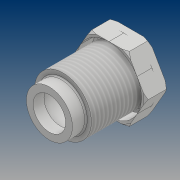
# Autodesk Inventor part: MUSAB2
Saved by Autodesk Inventor 2021 (Build 250183000, 183)
## iProperties
Created: 2017-09-12
Part Number: MUSAB2
Material: Generic
Document SubType Name: Modeling
Designer: Amer Mohia
Density: 1 g/cm^3
Appearance: Default
Author: Amer Mohia
Autodesk Inventor part; units mm, degrees
ref_plane "YZ Plane" through (0, 0, 0) normal (1, 0, 0) x (0, 1, 0)
ref_plane "XZ Plane" through (0, 0, 0) normal (0, 1, 0) x (-1, 0, 0)
sketch "Sketch1" plane through (0, 0, 0) normal (0, 0, 1) x (1, 0, 0)
  line L0 (-7.9743, 17.1273) -> (-7.9743, -10.9738)
  line L1 (4.0257, 11.5) -> (4.0257, 9)
  line L2 (4.0257, 9) -> (2.5257, 9)
  line L3 (2.5257, 9) -> (2.5257, -13.5)
  line L4 (2.5257, -13.5) -> (0.5257, -13.5)
  line L5 (0.5257, -13.5) -> (0.5257, -18.5)
  line L6 (4.0257, 11.5) -> (0.5257, 11.5)
  line L7 (0.5257, 11.5) -> (0.5257, 6.5)
  line L8 (0.5257, -2.5) -> (-0.9743, -2.5)
  line L9 (-0.9743, -2.5) -> (-0.9743, -11.3304)
  line L10 (-1.9743, -14.5) -> (-1.9743, -18.5)
  line L11 (-1.9743, -18.5) -> (0.5257, -18.5)
  line L12 (-1.9743, -14.5) -> (-0.9743, -14.5)
  line L13 (-0.9743, -14.5) -> (-0.9743, -11.3304)
  line L14 (0.0257, 6.5) -> (0.0257, 0)
  line L15 (0.5257, 6.5) -> (0.0257, 6.5)
  line L16 (0.0257, 0) -> (0.3257, 0)
  line L17 (0.8257, -0.5) -> (0.8257, -2.5)
  line L18 (0.8257, -2.5) -> (0.5257, -2.5)
  arc A0 (0.8257, -0.5) -> (0.3257, 0) centre (0.3257, -0.5) ccw
  point P0 (0.8257, 0)
  dimension "d6" = 14
  dimension "d7" = 17
  dimension "d8" = 21
  dimension "d10" = 5
  dimension "d11" = 12
  dimension "d12" = 4
  dimension "d13" = 30
  dimension "d14" = 5
  dimension "d18" = 24
  dimension "d19" = 16
  dimension "d20" = 17
  dimension "d21" = 0.8
  dimension "d22" = 2.5
  dimension "d23" = 0.5
  constraints: 38 end point, 8 perpendicular, 5 horizontal, 4 vertical, 3 point on line, 2 point on circle, 2 tangent, 1 centre point
  measures "d6" diameter of L9 L0
  measures "d7" diameter of L5 L0
  measures "d8" diameter of L3 L0
  measures "d10" distance of L4.end L5.end
  measures "d11" diameter of L10 L0
  measures "d12" distance of L10.start L10.end
  measures "d13" distance between parallel lines of L11 L6
  measures "d14" distance of L6.end L7.end
  measures "d18" diameter of L1 L0
  measures "d19" diameter of L14 L0
  measures "d20" diameter of L7 L0
  measures "d21" distance of L14.end point (0.826, 0)
  measures "d22" distance of point (0.826, 0) L17.end
  measures "d23" radius of A0
revolve "Revolution1" add sketch "Sketch1" angle 360 about axis through (-7.9743, 17.1273, 0) along (0, -1, 0)
sketch "Sketch2" plane through (-7.9743, 11.5, 0) normal (0, 1, 0) x (1, 0, 0)
  circle A0 centre (0, 0) radius 12 projected
  line L0 (6.9282, 12) -> (13.8564, 0)
  line L1 (13.8564, 0) -> (6.9282, -12)
  line L2 (6.9282, -12) -> (-6.9282, -12)
  line L3 (-6.9282, -12) -> (-13.8564, 0)
  line L4 (-13.8564, 0) -> (-6.9282, 12)
  line L5 (-6.9282, 12) -> (6.9282, 12)
  point P0 (7.9743, 0)
  point P1 (0, 12)
  constraints: 12 end point, 1 midpoint, 1 vertical alignment, 14 other
extrude "Extrusion1" add sketch "Sketch2" against normal blind 8 contours A0 L0 L1 | A0 L5 L0 | L1 L2 A0 | A0 L4 L5 | L2 L3 A0 | A0 L3 L4
sketch "Sketch3" plane through (0, 0, 0) normal (0, 0, 1) x (1, 0, 0)
  line L0 (2.418, 3.5) -> (5.8821, 3.5) projected
  line L1 (-1.0461, 11.5) -> (-1.0461, 3.5) projected
  line L2 (-1.0461, 11.5) -> (5.8821, 11.5) projected
  line L3 (5.8821, 11.5) -> (5.8821, 3.5) projected
  line L4 (-21.8307, 3.5) -> (-18.3666, 3.5) projected
  line L5 (-21.8307, 11.5) -> (-21.8307, 3.5) projected
  line L6 (-21.8307, 11.5) -> (-14.9025, 11.5) projected
  line L7 (-14.9025, 11.5) -> (-14.9025, 3.5) projected
  line L8 (-7.9743, 20.7963) -> (-7.9743, 13.4843)
  line L9 (6.3821, 12) -> (4.1894, 12)
  line L10 (6.3821, 12) -> (6.3821, 10.5)
  line L11 (4.1894, 12) -> (6.3821, 10.5)
  line L12 (-18.3666, 9) -> (-18.3666, 3.5) projected
  line L13 (-18.3666, 3.5) -> (-14.9025, 3.5) projected
  line L14 (2.418, 9) -> (2.418, 3.5) projected
  line L15 (-1.0461, 3.5) -> (2.418, 3.5) projected
  point P0 (0, 0)
  dimension "d36" = 0.5
  dimension "d38" = 0.5
  dimension "d39" = 1.5
  constraints: 8 end point, 2 vertical, 1 horizontal
  measures "d36" distance between parallel lines of L3 L10
  measures "d38" distance between parallel lines of L2 L9
  measures "d39" distance of L9.start L10.end
revolve "Revolution2" cut sketch "Sketch3" angle 360 about axis through (-7.9743, 20.7963, 0) along (0, -1, 0) contours L11 L2 L3 | L3 L2 L11 L9 L10
sketch "Sketch5" plane through (0, 0, 0) normal (0, 0, 1) x (1, 0, 0)
  point P0 (0, 0)
ref_plane "Work Plane2" through (-12.6935, 7.5, -12) normal (0, 1, 0) x (1, 0, 0)
mirror "Mirror2" about plane through (-12.6935, 7.5, -12) normal (0, 1, 0) of "Revolution2"
thread "Thread1" size "M16x0.75" class "6H" standard "ANSI Metric M Profile" length 9
thread "Thread2" size "M22x1.5" class "6g" standard "ANSI Metric M Profile" full length
fillet "Fillet1" radius 0.5 1 edges at (-16.4743, -13.5, 0)
fillet "Fillet2" radius 0.5 1 edges at (-18.4743, 9, 0)
body "Solid1"
